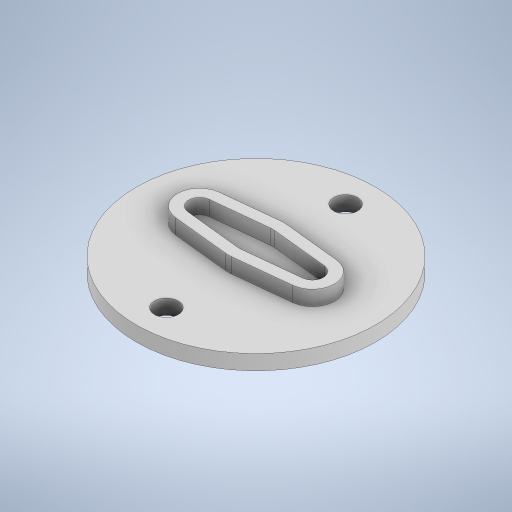
# Autodesk Inventor part: Rotating Disc
Saved by Autodesk Inventor 2024 (Build 280153000, 153)
## iProperties
Created: 2023-04-24
Part Number: Rotating Disc
Material: Generic
Document SubType Name: Modeling
Designer: byrne
Density: 1 g/cm^3
Appearance: Default
Author: byrne
Autodesk Inventor part; units mm, degrees
ref_plane "YZ Plane" through (0, 0, 0) normal (1, 0, 0) x (0, 1, 0)
ref_plane "XZ Plane" through (0, 0, 0) normal (0, 1, 0) x (-1, 0, 0)
ref_plane "XY Plane" through (0, 0, 0) normal (0, 0, 1) x (1, 0, 0)
sketch "Sketch1" plane through (0, 0, 0) normal (0, 1, 0) x (-1, 0, 0)
  circle A0 centre (0, 0) radius 25.4
  circle A1 centre (0, 19.05) radius 2.54
  circle A2 centre (0, -19.05) radius 2.54
  line L0 (0, 19.05) -> (0, -19.05) construction
  dimension "d0" = 50.8
  dimension "d1" = 5.08
  dimension "d2" = 5.08
  dimension "d3" = 38.1
  constraints: 3 centre point, 2 coincident, 2 end point, 1 midpoint, 1 vertical
  measures "d0" diameter of A0
  measures "d1" diameter of A1
  measures "d2" diameter of A2
  measures "d3" distance of L0.start L0.end
extrude "Extrusion1" add sketch "Sketch1" along normal blind 3.175
sketch "Sketch2" plane through (0, 3.175, 0) normal (0, 1, 0) x (1, 0, 0)
  circle A0 centre (0, 0) radius 2.75
  circle A1 centre (-12, 0) radius 1.5
  circle A2 centre (12, 0) radius 1.5
  line L0 (-12, 0) -> (12, 0) construction
  line L1 (-12.1563, 1.4918) -> (-0.2865, 2.735)
  line L2 (0.2865, -2.735) -> (12.1563, -1.4918)
  line L3 (0.2865, 2.735) -> (12.1562, 1.4918)
  line L4 (-0.2865, -2.735) -> (-12.1563, -1.4918)
  circle A3 centre (-12, 0) radius 2.2938
  line L5 (-12.2389, 2.2813) -> (-0.3691, 3.5245)
  line L6 (-0.3691, -3.5245) -> (-12.2389, -2.2813)
  circle A4 centre (0, 0) radius 3.5438
  line L7 (0.3691, 3.5245) -> (12.2389, 2.2813)
  line L8 (0.3691, -3.5245) -> (12.2389, -2.2813)
  circle A5 centre (12, 0) radius 2.2938
  line L9 (0.6172, -5.8928) -> (12.487, -4.6496)
  circle A6 centre (12, 0) radius 4.675
  line L10 (0.6172, 5.8928) -> (12.487, 4.6496)
  circle A7 centre (0, 0) radius 5.925
  line L11 (-12.487, 4.6496) -> (-0.6172, 5.8928)
  line L12 (-0.6172, -5.8928) -> (-12.487, -4.6496)
  circle A8 centre (-12, 0) radius 4.675
  point P0 (-0.3691, 3.5245)
  point P1 (-0.6172, 5.8928)
  dimension "d6" = 5.5
  dimension "d7" = 3
  dimension "d8" = 27
  dimension "d9" = 0.7937
  dimension "d10" = 0.7937
  dimension "d11" = 0.7937
  dimension "d12" = 0.7937
  dimension "d13" = 0.7937
  dimension "d14" = 0.7937
  dimension "d15" = 0.7937
  dimension "d16" = 2.3813
  dimension "d17" = 2.3813
  dimension "d18" = 2.3813
  dimension "d19" = 2.3813
  dimension "d20" = 2.3813
  dimension "d21" = 2.3813
  dimension "d22" = 2.3813
  constraints: 26 end point, 9 centre point, 9 parallel, 8 point on circle, 7 tangent, 2 coincident, 1 equal radius, 1 horizontal, 1 midpoint
  measures "d6" diameter of A0
  measures "d7" diameter of A1
  measures "d9" radial gap between concentric circles of A1 A3
  measures "d10" distance between parallel lines of L1 L5
  measures "d11" distance between parallel lines of L4 L6
  measures "d12" radial gap between concentric circles of A0 A4
  measures "d13" distance between parallel lines of L3 L7
  measures "d14" distance between parallel lines of L2 L8
  measures "d15" radial gap between concentric circles of A2 A5
  measures "d16" distance between parallel lines of L8 L9
  measures "d17" radial gap between concentric circles of A5 A6
  measures "d18" distance between parallel lines of L7 L10
  measures "d19" radial gap between concentric circles of A4 A7
  measures "d20" distance between parallel lines of L5 L11
  measures "d21" distance between parallel lines of L6 L12
  measures "d22" radial gap between concentric circles of A3 A8
extrude "Extrusion2" add sketch "Sketch2" along normal blind 3.175 contours A4 L5 A7 L7 | L8 A7 L6 A4 | A7 L10 A6 L7 | L8 A6 L9 A7 | L5 A8 L11 A7 | A6 L8 A5 L7 | A7 L12 A8 L6 | L5 A3 L6 A8
equation "\"d9\" = d11"
equation "\"d10\" = d14"
equation "\"d11\" = d14"
equation "\"d12\" = d11"
equation "\"d13\" = d14"
equation "\"d15\" = d14"
equation "\"d17\" = d16"
equation "\"d18\" = d16"
equation "\"d19\" = d16"
equation "\"d20\" = d16"
equation "\"d21\" = d16"
equation "\"d22\" = d16"
body "Solid1"
